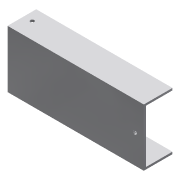
# Autodesk Inventor part: U profil
Saved by Autodesk Inventor 2015 (Build 190159000, 159)
## iProperties
Created: 2015-01-07
Part Number: U profil
Material: Všeobecné
Document SubType Name: Modeling
Designer: Michal
Density: 1 g/cm^3
Appearance: Hliník – leštěný
Author: Michal
Autodesk Inventor part; units mm, degrees
ref_plane "YZ Plane" through (0, 0, 0) normal (1, 0, 0) x (0, 1, 0)
ref_plane "XZ Plane" through (0, 0, 0) normal (0, 1, 0) x (-1, 0, 0)
ref_plane "XY Plane" through (0, 0, 0) normal (0, 0, 1) x (1, 0, 0)
sketch "Náčrt1" plane through (0, 0, 0) normal (1, 0, 0) x (0, 1, 0)
  line L0 (0, 0) -> (80, 0)
  line L1 (80, 0) -> (80, -6)
  line L2 (80, -6) -> (6, -6)
  line L3 (6, -6) -> (6, -154)
  line L4 (6, -154) -> (80, -154)
  line L5 (80, -154) -> (80, -160)
  line L6 (80, -160) -> (0, -160)
  line L7 (0, -160) -> (0, 0)
  dimension "d0" = 80
  dimension "d1" = 6
  dimension "d3" = 148
  dimension "d5" = 6
  dimension "d6" = 80
  dimension "d20" = 160
  dimension "d21" = 74
  constraints: 16 end point, 4 perpendicular, 2 point on line, 1 horizontal
  measures "d0" distance of L0.start L0.end
  measures "d1" distance of L0.end L1.end
  measures "d3" distance of L2.end L3.end
  measures "d5" distance of L4.end L5.end
  measures "d6" distance of L5.end L6.end
  measures "d20" distance of L6.end L0.start
  measures "d21" distance of L1.end L2.end
extrude "Vysunutí1" add sketch "Náčrt1" along normal blind 380
sketch "Náčrt4" plane through (0, 6, -6) normal (0, 1, 0) x (1, 0, 0)
  line L0 (0, 0) -> (0, 148) projected
  line L1 (0, 0) -> (380, 0) projected
  line L2 (380, 148) -> (380, 0) projected
  line L3 (0, 148) -> (380, 148) projected
  circle A0 centre (355, 74) radius 5.25
  line L4 (0, 154) -> (380, 154) projected
  point P0 (0, -6)
  dimension "d14" = 25
  dimension "d15" = 80
  dimension "d16" = 10.5
  constraints: 1 centre point
  measures "d14" distance from line of L2 A0.centre
  measures "d15" distance from line of L4 A0.centre
  measures "d16" diameter of A0
extrude "Vysunutí3" cut sketch "Náčrt4" against normal through all contours A0
sketch "Náčrt5" plane through (0, 0, 0) normal (0, 0, 1) x (1, 0, 0)
  circle A0 centre (23, 46) radius 5.25
  line L0 (380, 80) -> (380, 0) projected
  line L1 (0, 0) -> (380, 0) projected
  dimension "d22" = 10.5
  dimension "d23" = 357
  dimension "d24" = 46
  constraints: 1 centre point
  measures "d22" diameter of A0
  measures "d23" distance from line of L0 A0.centre
  measures "d24" distance from line of L1 A0.centre
extrude "Vysunutí4" cut sketch "Náčrt5" against normal through all
sketch "Náčrt6" plane through (0, 0, -160) normal (0, 0, -1) x (-1, 0, 0)
  circle A0 centre (-23, 46) radius 5.25 projected
  line L0 (0, 80) -> (0, 0) projected
  line L1 (0, 80) -> (-380, 80) projected
  line L2 (-380, 0) -> (-380, 80) projected
  line L3 (0, 0) -> (-380, 0) projected
  line L4 (-219.2388, 40) -> (-154.125, 40)
  line L5 (-190, 7.0383) -> (-190, 75.4408)
  arc A1 (-216.8837, 45.7895) -> (-209.5518, 44.2105) centre (-213.2177, 45) ccw
  arc A2 (-209.5518, 35.7895) -> (-216.8837, 34.2105) centre (-213.2177, 35) ccw
  arc A3 (-195.7895, 13.1163) -> (-194.2105, 20.4482) centre (-195, 16.7823) ccw
  arc A4 (-185.7895, 20.4482) -> (-184.2105, 13.1163) centre (-185, 16.7823) ccw
  arc A5 (-163.1163, 34.2105) -> (-170.4482, 35.7895) centre (-166.7823, 35) ccw
  arc A6 (-170.4482, 44.2105) -> (-163.1163, 45.7895) centre (-166.7823, 45) ccw
  arc A7 (-184.2105, 66.8837) -> (-185.7895, 59.5518) centre (-185, 63.2177) ccw
  arc A8 (-194.2105, 59.5518) -> (-195.7895, 66.8837) centre (-195, 63.2177) ccw
  arc A9 (-194.2105, 59.5518) -> (-209.5518, 44.2105) centre (-190, 40) ccw
  arc A10 (-195.7895, 66.8837) -> (-216.8837, 45.7895) centre (-190, 40) ccw
  arc A11 (-163.1163, 45.7895) -> (-184.2105, 66.8837) centre (-190, 40) ccw
  arc A12 (-170.4482, 44.2105) -> (-185.7895, 59.5518) centre (-190, 40) ccw
  arc A13 (-216.8837, 34.2105) -> (-195.7895, 13.1163) centre (-190, 40) ccw
  arc A14 (-184.2105, 13.1163) -> (-163.1163, 34.2105) centre (-190, 40) ccw
  arc A15 (-209.5518, 35.7895) -> (-194.2105, 20.4482) centre (-190, 40) ccw
  arc A16 (-185.7895, 20.4482) -> (-170.4482, 35.7895) centre (-190, 40) ccw
  point P0 (0, 0)
  dimension "d22" = 10.5
  dimension "d29" = 190
  dimension "d30" = 40
  dimension "d31" = 5
  dimension "d32" = 5
  dimension "d35" = 360
  constraints: 32 point on circle, 16 centre point, 4 end point, 2 coincident, 1 horizontal, 1 point on line, 1 vertical, 33 other
  measures "d29" distance from line of L0 A10.centre
  measures "d30" distance from line of L1 A10.centre
  measures "d31" distance from line of L4 A1.centre
  measures "d32" distance from line of L4 A2.centre
extrude "Vysunutí5" cut sketch "Náčrt6" against normal up to surface (6 mm away) contours A10 A8 A9 A1 | A15 A3 A13 A2 | A16 A5 A14 A4 | A12 A7 A11 A6
